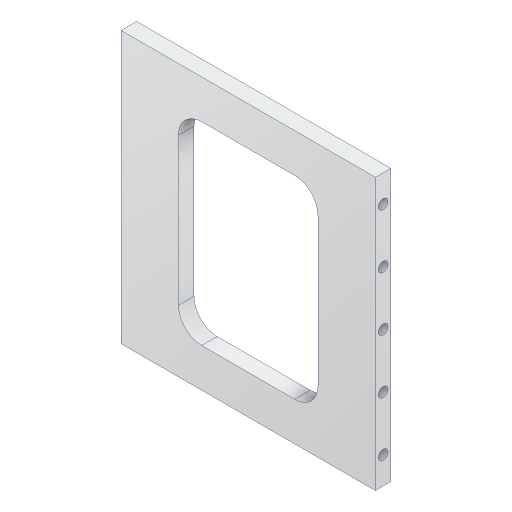
# Autodesk Inventor part: 지지프레임2
Saved by Autodesk Inventor 2023.2 (Build 272271000, 271)
## iProperties
Created: 2022-12-28
Part Number: 지지프레임2
Material: 알루미늄 6061
Document SubType Name: Modeling
Designer: BAEK
Density: 2.7 g/cm^3
Appearance: 알루미늄 - 평지
Mass: 22.8665 g
Surface Area: 63.4784 cm^2
Volume: 8.46909 cm^3
Author: BAEK
Autodesk Inventor part; units mm, degrees
ref_plane "YZ Plane" through (0, 0, 0) normal (1, 0, 0) x (0, 1, 0)
ref_plane "XZ Plane" through (0, 0, 0) normal (0, 1, 0) x (-1, 0, 0)
ref_plane "XY Plane" through (0, 0, 0) normal (0, 0, 1) x (1, 0, 0)
sketch "스케치1" plane through (0, 0, 0) normal (0, 0, 1) x (1, 0, 0)
  line L0 (-32.8, 35) -> (32.8, 35)
  line L1 (32.8, 35) -> (32.8, -35)
  line L2 (32.8, -35) -> (-32.8, -35)
  line L3 (-32.8, -35) -> (-32.8, 35)
  line L4 (-32.8, 35) -> (32.8, -35) construction
  line L5 (32.8, 35) -> (-32.8, -35) construction
  point P0 (0, 0)
  dimension "d0" = 65.6
  dimension "d1" = 70
  constraints: 12 end point, 2 midpoint, 2 parallel, 1 horizontal, 1 perpendicular
  measures "d0" distance of L1.end L2.end
  measures "d1" distance of L0.end L1.end
extrude "돌출1" add sketch "스케치1" along normal blind 4
sketch "스케치2" plane through (32.8, -35, 0) normal (1, 0, 0) x (0, 0, -1)
  line L0 (0, 0) -> (0, 70) projected
  line L1 (0, 70) -> (-4, 70) projected
  line L2 (-4, 0) -> (-4, 70) projected
  line L3 (0, 0) -> (-4, 0) projected
  line L4 (0, 70) -> (-4, 70) projected
  line L5 (-2, 70) -> (-2, 0) construction
  line L6 (0, 0) -> (-4, 0) projected
  circle A0 centre (-2, 63) radius 1.25
  circle A1 centre (-2, 49) radius 1.25
  circle A2 centre (-2, 35) radius 1.25
  circle A3 centre (-2, 21) radius 1.25
  circle A4 centre (-2, 7) radius 1.25
  point P0 (0, 35)
  dimension "d4" = 2.5
  dimension "d5" = 2.5
  dimension "d6" = 2.5
  dimension "d8" = 2.5
  dimension "d9" = 2.5
  dimension "d10" = 14
  dimension "d11" = 7
  dimension "d12" = 14
  dimension "d13" = 7
  dimension "d14" = 14
  constraints: 5 centre point, 4 midpoint, 4 point on line, 2 end point
  measures "d4" diameter of A0
  measures "d5" diameter of A1
  measures "d6" diameter of A2
  measures "d8" diameter of A3
  measures "d9" diameter of A4
  measures "d10" distance of A0.centre A1.centre
  measures "d11" distance from line of L4 A0.centre
  measures "d12" distance of A1.centre A2.centre
  measures "d13" distance of point (-2, 0) A4.centre
  measures "d14" distance of A4.centre A3.centre
extrude "돌출2" cut sketch "스케치2" against normal blind 6 contours A0 | A1 | A2 | A3 | A4
mirror "미러1" about plane through (0, 0, 0) normal (1, 0, 0) of "돌출2"
sketch "스케치3" plane through (0, 0, 0) normal (0, 0, -1) x (-1, 0, 0)
  line L0 (-18, 25) -> (18, 25)
  line L1 (18, 25) -> (18, -25)
  line L2 (18, -25) -> (-18, -25)
  line L3 (-18, -25) -> (-18, 25)
  line L4 (-18, 25) -> (18, -25) construction
  line L5 (18, 25) -> (-18, -25) construction
  point P0 (0, 0)
  dimension "d19" = 36
  dimension "d20" = 50
  constraints: 12 end point, 2 midpoint, 2 parallel, 1 horizontal, 1 perpendicular
  measures "d19" distance of L1.end L2.end
  measures "d20" distance of L0.end L1.end
extrude "돌출3" cut sketch "스케치3" against normal blind 6
fillet "모깎기1" radius 6 4 edges at (18, 25, 2) (-18, 25, 2) (-18, -25, 2) (18, -25, 2)
